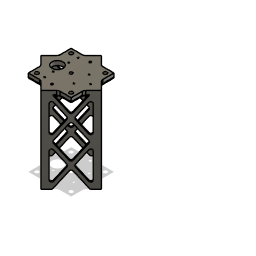
sensors-plate_lidar3d_generic-support (Autodesk Fusion 360 design; units mm, degrees)
Autodesk Fusion 360 part; units mm, degrees
note: some values were not read from the file. Set by a fixed rule: which sketch regions a step uses.
ref_plane "WorkPlane1" through (176, 592, -131) normal (0, 1, 0) x (-1, 0, 0)
sketch "Sketch4" plane through (0, 592, 0) normal (0, 1, 0) x (1, 0, 0)
  line L0 (178, -131) -> (180, -131)
  line L1 (176, 131) -> (178, 131)
  line L2 (176, -131) -> (178, -131)
  line L3 (178, 131) -> (180, 131)
  line L4 (180, -131) -> (180, 131)
  line L5 (176, 133) -> (176, 135)
  line L6 (-176, 131) -> (-176, 133)
  line L7 (176, 131) -> (176, 133)
  line L8 (-176, 133) -> (-176, 135)
  line L9 (176, 135) -> (-176, 135)
  line L10 (-176, -133) -> (-176, -135)
  line L11 (176, -131) -> (176, -133)
  line L12 (-176, -131) -> (-176, -133)
  line L13 (176, -133) -> (176, -135)
  line L14 (-176, -135) -> (176, -135)
  line L15 (-178, 131) -> (-180, 131)
  line L16 (-176, -131) -> (-178, -131)
  line L17 (-176, 131) -> (-178, 131)
  line L18 (-178, -131) -> (-180, -131)
  line L19 (-180, 131) -> (-180, -131)
  circle A0 centre (-120, 60) radius 2 construction
  circle A1 centre (0, -120) radius 2 construction
  circle A2 centre (-120, -120) radius 2 construction
  circle A3 centre (120, 0) radius 2 construction
  circle A4 centre (0, 120) radius 2 construction
  circle A5 centre (0, 60) radius 2 construction
  circle A6 centre (-165.5, -26.5835) radius 2.5
  circle A7 centre (0, 0) radius 2 construction
  circle A8 centre (-60, -120) radius 2 construction
  circle A9 centre (165.5, 26.5835) radius 2.5
  circle A10 centre (-165.5, -78.1855) radius 2.5
  circle A11 centre (-120, 0) radius 2 construction
  circle A12 centre (-120, 120) radius 2 construction
  circle A13 centre (60, -60) radius 2 construction
  circle A14 centre (60, -120) radius 2 construction
  circle A15 centre (120, 60) radius 2 construction
  circle A16 centre (-60, -60) radius 2 construction
  circle A17 centre (0, -60) radius 2 construction
  circle A18 centre (-165.5, 26.5835) radius 2.5
  circle A19 centre (-60, 60) radius 2 construction
  circle A20 centre (165.5, -26.5835) radius 2.5
  circle A21 centre (-60, 0) radius 2 construction
  circle A22 centre (-120, -60) radius 2 construction
  circle A23 centre (-165.5, 78.1855) radius 2.5
  circle A24 centre (120, -60) radius 2 construction
  circle A25 centre (120, -120) radius 2 construction
  circle A26 centre (60, 120) radius 2 construction
  circle A27 centre (165.5, -78.1855) radius 2.5
  circle A28 centre (120, 120) radius 2 construction
  circle A29 centre (60, 0) radius 2 construction
  circle A30 centre (-60, 120) radius 2 construction
  circle A31 centre (165.5, 78.1855) radius 2.5
  circle A32 centre (60, 60) radius 2 construction
  line L20 (0, 70.7107) -> (-70.7107, 0)
  line L21 (-70.7107, 0) -> (0, -70.7107)
  line L22 (0, -70.7107) -> (70.7107, 0)
  line L23 (70.7107, 0) -> (0, 70.7107)
  line L24 (-180, 0) -> (180, 0) construction
  dimension "d323" = 50
  dimension "d324" = 135
  constraint coincident A7.centre origin
  constraint midpoint L19 L24.start
  constraint midpoint L4 L24.end
  measures "d323" distance of A7.centre L23
  measures "d324" angle of L23 L24
extrude "Extrude2" add sketch "Sketch4" against normal blind 8 contours L20 L21 L22 L23
sketch "Sketch6" plane through (0, 584, 0) normal (0, -1, 0) x (1, 0, 0)
  line L0 (0, -70.7107) -> (70.7107, 0)
  line L1 (70.7107, 0) -> (0, 70.7107)
  line L2 (0, 70.7107) -> (-70.7107, 0)
  line L3 (-70.7107, 0) -> (0, -70.7107)
  line L4 (180, -131) -> (180, 131)
  line L5 (180, -131) -> (176, -131)
  line L6 (176, 131) -> (180, 131)
  line L7 (-176, -135) -> (176, -135)
  line L8 (-176, -135) -> (-176, -131)
  line L9 (176, -131) -> (176, -135)
  line L10 (176, 135) -> (-176, 135)
  line L11 (176, 135) -> (176, 131)
  line L12 (-176, 131) -> (-176, 135)
  line L13 (-180, 131) -> (-180, -131)
  line L14 (-180, 131) -> (-176, 131)
  line L15 (-176, -131) -> (-180, -131)
  circle A0 centre (-120, -60) radius 2
  circle A1 centre (0, 120) radius 2
  circle A2 centre (-120, 120) radius 2
  circle A3 centre (120, 0) radius 2
  circle A4 centre (0, -120) radius 2
  circle A5 centre (0, -60) radius 2 construction
  circle A6 centre (-165.5, 26.5835) radius 2.5
  circle A7 centre (0, 0) radius 2 construction
  circle A8 centre (-60, 120) radius 2
  circle A9 centre (165.5, -26.5835) radius 2.5
  circle A10 centre (-165.5, 78.1855) radius 2.5
  circle A11 centre (-120, 0) radius 2
  circle A12 centre (-120, -120) radius 2
  circle A13 centre (60, 60) radius 2
  circle A14 centre (60, 120) radius 2
  circle A15 centre (120, -60) radius 2
  circle A16 centre (-60, 60) radius 2
  circle A17 centre (0, 60) radius 2 construction
  circle A18 centre (-165.5, -26.5835) radius 2.5
  circle A19 centre (-60, -60) radius 2
  circle A20 centre (165.5, 26.5835) radius 2.5
  circle A21 centre (-60, 0) radius 2 construction
  circle A22 centre (-120, 60) radius 2
  circle A23 centre (-165.5, -78.1855) radius 2.5
  circle A24 centre (120, 60) radius 2
  circle A25 centre (120, 120) radius 2
  circle A26 centre (60, -120) radius 2
  circle A27 centre (165.5, 78.1855) radius 2.5
  circle A28 centre (120, -120) radius 2
  circle A29 centre (60, 0) radius 2 construction
  circle A30 centre (-60, -120) radius 2
  circle A31 centre (165.5, -78.1855) radius 2.5
  circle A32 centre (60, -60) radius 2
  line L16 (45, 0) -> (-22.5, 38.9711) construction
  line L17 (-22.5, 38.9711) -> (-22.5, -38.9711) construction
  line L18 (-22.5, -38.9711) -> (45, 0) construction
  line L19 (45, 0) -> (-22.5, 0) construction
  line L20 (-70.7107, 0) -> (70.7107, 0) construction
  line L21 (0, 70.7107) -> (0, -70.7107) construction
  circle A33 centre (-22.5, 38.9711) radius 1.65
  circle A34 centre (45, 0) radius 1.65
  circle A35 centre (-22.5, -38.9711) radius 1.65
  line L22 (40, 40) -> (-40, 40) construction
  line L23 (-40, 40) -> (-40, -40) construction
  line L24 (-40, -40) -> (40, -40) construction
  line L25 (40, -40) -> (40, 40) construction
  circle A36 centre (-40, 40) radius 4.15
  circle A37 centre (40, 40) radius 4.15
  circle A38 centre (40, -40) radius 4.15
  circle A39 centre (-40, -40) radius 4.15
  line L26 (50, 50) -> (-50, 50)
  line L27 (-50, 50) -> (-50, -50)
  line L28 (-50, -50) -> (50, -50)
  line L29 (50, -50) -> (50, 50)
  circle A40 centre (-24, 18) radius 1.65
  circle A41 centre (24, 18) radius 1.65
  circle A42 centre (24, -18) radius 1.65
  circle A43 centre (-24, -18) radius 1.65
  circle A44 centre (0, 0) radius 3.325
  circle A45 centre (0, 44.45) radius 2.15
  circle A46 centre (0, -44.45) radius 2.15
  circle A47 centre (0, 0) radius 45 construction
  circle A48 centre (0, -45) radius 2.15
  circle A49 centre (0, 45) radius 2.15
  line L30 (-2.15, -44.45) -> (-2.15, -45)
  line L31 (2.15, -44.45) -> (2.15, -45)
  line L32 (-2.15, 44.45) -> (-2.15, 45)
  line L33 (2.15, 45) -> (2.15, 44.45)
  circle A50 centre (0, 0) radius 24 construction
  circle A51 centre (0, 0) radius 40 construction
  circle A52 centre (-32, 0) radius 8 construction
  circle A53 centre (-32, 0) radius 13
  line L34 (-60, 0) -> (0, 60) construction
  line L35 (0, 60) -> (60, 0) construction
  line L36 (60, 0) -> (0, -60) construction
  line L37 (0, -60) -> (-60, 0) construction
  line L38 (-51.5147, 0) -> (0, 51.5147) construction
  line L39 (0, 51.5147) -> (51.5147, 0) construction
  line L40 (51.5147, 0) -> (0, -51.5147) construction
  line L41 (0, -51.5147) -> (-51.5147, 0) construction
  line L42 (-51.5147, 0) -> (-61.1127, 9.598)
  line L43 (-51.5147, 0) -> (-61.1127, -9.598)
  line L44 (0, 51.5147) -> (9.598, 61.1127)
  line L45 (0, 51.5147) -> (-9.598, 61.1127)
  line L46 (0, -51.5147) -> (-9.598, -61.1127)
  line L47 (0, -51.5147) -> (9.598, -61.1127)
  line L48 (51.5147, 0) -> (61.1127, -9.598)
  line L49 (51.5147, 0) -> (61.1127, 9.598)
  dimension "d331" = 45
  dimension "d332" = 3.3
  dimension "d333" = 40
  dimension "d334" = 135
  dimension "d335" = 8.3
  dimension "d336" = 50
  dimension "d338" = 3.3
  dimension "d339" = 6.65
  dimension "d340" = 4.3
  dimension "d341" = 88.9
  dimension "d536" = 48
  dimension "d537" = 80
  dimension "d538" = 5
  dimension "d539" = 24
  dimension "d540" = 18
  dimension "d545" = 6
  constraint coincident A7.centre A44.centre
  constraint midpoint L17 L19.end
  constraint coincident L2.end L3.start
  constraint coincident L0.end L1.start
  constraint coincident L1.end L2.start
  constraint coincident L0.start L3.end
  constraint collinear L19 L20
  constraint coincident L16.end L17.start
  constraint coincident L16.start L18.end
  constraint coincident L17.end L18.start
  constraint equal A33 A35
  constraint equal A33 A34
  constraint coincident L22.end L23.start
  constraint coincident L22.start L25.end
  constraint coincident L24.end L25.start
  constraint coincident L23.end L24.start
  constraint equal A36 A39
  constraint equal A36 A38
  constraint equal A36 A37
  constraint parallel L25 L29
  constraint equal A40 A43
  constraint equal A40 A41
  constraint equal A40 A42
  constraint coincident L21 A45.centre
  constraint coincident L21 A46.centre
  constraint symmetric L20 A45 A46
  constraint coincident L16.start A47
  constraint coincident L21 A48.centre
  constraint coincident A47 A48.centre
  constraint coincident A47 A49.centre
  constraint coincident L21 A49.centre
  constraint equal A45 A49
  constraint equal A45 A48
  constraint coincident A46 L30.start
  constraint coincident A48 L30.end
  constraint coincident A46 L31.start
  constraint coincident A48 L31.end
  constraint tangent A46 L30
  constraint tangent A48 L30
  constraint tangent A46 L31
  constraint tangent A48 L31
  constraint coincident A45 L32.start
  constraint coincident A49 L32.end
  constraint coincident A49 L33.start
  constraint coincident A45 L33.end
  constraint tangent A49 L33
  constraint tangent A45 L33
  constraint tangent A49 L32
  constraint tangent A45 L32
  constraint concentric A44 A50
  constraint tangent A50 A52
  constraint tangent A51 A52
  constraint coincident L20 A52.centre
  constraint symmetric L21 A40 A41
  constraint symmetric L20 A40 A43
  constraint symmetric L20 A41 A42
  constraint coincident A21.centre L34.start
  constraint coincident A17.centre L34.end
  constraint coincident A29.centre L35.end
  constraint coincident A5.centre L36.end
  constraint coincident L2 L42.end
  constraint perpendicular L2 L42
  constraint coincident L3 L43.end
  constraint perpendicular L3 L43
  constraint coincident L1 L44.end
  constraint perpendicular L1 L44
  constraint coincident L2 L45.end
  constraint perpendicular L2 L45
  constraint coincident L3 L46.end
  constraint perpendicular L3 L46
  constraint coincident L0 L47.end
  constraint perpendicular L0 L47
  constraint coincident L0 L48.end
  constraint perpendicular L0 L48
  constraint coincident L1 L49.end
  constraint perpendicular L1 L49
  measures "d331" distance of L16.start A7.centre
  measures "d332" diameter of A33
  measures "d333" distance of A7.centre L25
  measures "d334" angle of L1 L25
  measures "d335" diameter of A36
  measures "d336" distance of A7.centre L29
  measures "d338" diameter of A40
  measures "d339" diameter of A44
  measures "d340" diameter of A45
  measures "d341" distance of A45.centre A46.centre
  measures "d536" diameter of A50
  measures "d537" diameter of A51
  measures "d539" distance of L21 A41.centre
  measures "d540" distance of L20 A41.centre
extrude "Extrude3" cut sketch "Sketch6" against normal up to surface (8 mm away) contours A33 | A34 | A35 | A40 | A41 | A42 | A43 | A44 | A45 A49 | A45 A49 L32 | A45 A49 L33 | A45 A49 | A45 A49 | A46 A48 | A46 A48 L31 | A46 A48 L30 | A46 A48 | A46 A48 | A53
extrude "Extrude4" add sketch "Sketch6" against normal up to surface (8 mm away) contours L0 L28 L29 | L3 L27 L28 | L1 L26 L29 | L2 L26 L27
extrude "Extrude5" add sketch "Sketch6" along normal up to surface (192 mm away) contours L0 L3 L46 L47 | L0 L1 L48 L49 | L2 L3 L42 L43 | L1 L2 L44 L45
sketch "Sketch7" plane through (-35.3553, 0, -35.3553) normal (-0.707107, 0, -0.707107) x (-0.707107, 0, 0.707107)
  line L0 (20.7107, 592) -> (20.7107, 584)
  line L1 (20.7107, 584) -> (36.4264, 584)
  line L2 (36.4264, 584) -> (36.4264, 392)
  line L3 (36.4264, 392) -> (50, 392)
  line L4 (50, 392) -> (50, 592)
  line L5 (50, 592) -> (20.7107, 592)
  line L6 (-20.7107, 584) -> (-20.7107, 592)
  line L7 (-20.7107, 592) -> (-50, 592)
  line L8 (-50, 592) -> (-50, 392)
  line L9 (-50, 392) -> (-36.4264, 392)
  line L10 (-36.4264, 392) -> (-36.4264, 584)
  line L11 (-36.4264, 584) -> (-20.7107, 584)
  line L12 (36.4264, 584) -> (-36.4264, 488) construction
  line L13 (-36.4264, 488) -> (36.4264, 392) construction
  line L14 (-36.4264, 392) -> (36.4264, 488) construction
  line L15 (36.4264, 488) -> (-36.4264, 584) construction
  line L16 (-33.24, 389.5819) -> (41.4478, 488)
  line L17 (41.4478, 488) -> (-33.24, 586.4181)
  line L18 (-39.6128, 394.4181) -> (31.405, 488)
  line L19 (31.405, 488) -> (-39.6128, 581.5819)
  line L20 (33.24, 586.4181) -> (-41.4478, 488)
  line L21 (-41.4478, 488) -> (33.24, 389.5819)
  line L22 (39.6128, 581.5819) -> (-31.405, 488)
  line L23 (-31.405, 488) -> (39.6128, 394.4181)
  line L24 (36.4264, 392) -> (-36.4264, 392)
  dimension "d549" = 4
  dimension "d550" = -4
  dimension "d551" = 4
  dimension "d552" = -4
  constraint coincident L1.end L2.start
  constraint midpoint L10 L12.end
  constraint coincident L2.end L3.start
  constraint coincident L9.end L10.start
  constraint midpoint L2 L14.end
  constraint coincident L10.end L11.start
extrude "Extrude6" add sketch "Sketch7" against normal blind 4 contours L1 L2 L17 L20 L22 | L10 L11 L17 L19 L20 | L17 L19 L20 L22 | L2 L16 L21 L23 L24 | L2 L16 L17 L18 L19 L22 L23 | L10 L18 L19 L20 L21 L22 L23 | L16 L18 L21 L23 | L10 L16 L18 L21 L24
sketch "Sketch8" plane through (35.3553, 0, 35.3553) normal (0.707107, 0, 0.707107) x (0.707107, 0, -0.707107)
  line L0 (-20.7107, 584) -> (-20.7107, 592)
  line L1 (-20.7107, 592) -> (-50, 592)
  line L2 (-50, 592) -> (-50, 392)
  line L3 (-50, 392) -> (-36.4264, 392)
  line L4 (-36.4264, 392) -> (-36.4264, 584)
  line L5 (-36.4264, 584) -> (-20.7107, 584)
  line L6 (31.405, 488) -> (0, 446.6168)
  line L7 (0, 446.6168) -> (-31.405, 488)
  line L8 (-31.405, 488) -> (0, 529.3832)
  line L9 (0, 529.3832) -> (31.405, 488)
  line L10 (-36.4264, 481.3832) -> (-5.0214, 440)
  line L11 (-5.0214, 440) -> (-36.4264, 398.6168)
  line L12 (-36.4264, 398.6168) -> (-36.4264, 392)
  line L13 (-36.4264, 392) -> (-31.405, 392)
  line L14 (-31.405, 392) -> (0, 433.3832)
  line L15 (0, 433.3832) -> (31.405, 392)
  line L16 (31.405, 392) -> (36.4264, 392)
  line L17 (36.4264, 392) -> (36.4264, 398.6168)
  line L18 (36.4264, 398.6168) -> (5.0214, 440)
  line L19 (5.0214, 440) -> (36.4264, 481.3832)
  line L20 (36.4264, 481.3832) -> (36.4264, 494.6168)
  line L21 (36.4264, 494.6168) -> (5.0214, 536)
  line L22 (5.0214, 536) -> (36.4264, 577.3832)
  line L23 (36.4264, 577.3832) -> (36.4264, 584)
  line L24 (36.4264, 584) -> (31.405, 584)
  line L25 (31.405, 584) -> (0, 542.6168)
  line L26 (0, 542.6168) -> (-31.405, 584)
  line L27 (-31.405, 584) -> (-36.4264, 584)
  line L28 (-36.4264, 584) -> (-36.4264, 577.3832)
  line L29 (-36.4264, 577.3832) -> (-5.0214, 536)
  line L30 (-5.0214, 536) -> (-36.4264, 494.6168)
  line L31 (-36.4264, 494.6168) -> (-36.4264, 481.3832)
extrude "Extrude7" add sketch "Sketch8" against normal blind 4 contours L4 L5 L10 L11 L12 L13 L14 L15 L16 L17 L18 L19 L20 L21 L22 L23 L24 L25 L26 L27 L28 L29 L30 L31
sketch "Sketch9" plane through (-35.3553, 0, 35.3553) normal (-0.707107, 0, 0.707107) x (0.707107, 0, 0.707107)
  line L0 (-20.7107, 584) -> (-20.7107, 592)
  line L1 (-20.7107, 592) -> (-50, 592)
  line L2 (-50, 592) -> (-50, 392)
  line L3 (-50, 392) -> (-36.4264, 392)
  line L4 (-36.4264, 392) -> (-36.4264, 584)
  line L5 (-36.4264, 584) -> (-20.7107, 584)
  line L6 (20.7107, 592) -> (20.7107, 584)
  line L7 (20.7107, 584) -> (36.4264, 584)
  line L8 (36.4264, 584) -> (36.4264, 392)
  line L9 (36.4264, 392) -> (50, 392)
  line L10 (50, 392) -> (50, 592)
  line L11 (50, 592) -> (20.7107, 592)
  line L12 (-36.4264, 584) -> (36.4264, 488) construction
  line L13 (36.4264, 488) -> (-36.4264, 392) construction
  line L14 (36.4264, 392) -> (-36.4264, 488) construction
  line L15 (-36.4264, 488) -> (36.4264, 584) construction
  line L16 (39.6128, 394.4181) -> (-31.405, 488)
  line L17 (-31.405, 488) -> (39.6128, 581.5819)
  line L18 (33.24, 389.5819) -> (-41.4478, 488)
  line L19 (-41.4478, 488) -> (33.24, 586.4181)
  line L20 (-39.6128, 581.5819) -> (31.405, 488)
  line L21 (31.405, 488) -> (-39.6128, 394.4181)
  line L22 (-33.24, 586.4181) -> (41.4478, 488)
  line L23 (41.4478, 488) -> (-33.24, 389.5819)
  line L24 (36.4264, 392) -> (-36.4264, 392)
  dimension "d557" = 4
  dimension "d558" = -4
  dimension "d559" = 4
  dimension "d560" = -4
  constraint coincident L4.end L5.start
  constraint midpoint L8 L12.end
  constraint coincident L3.end L4.start
  constraint coincident L8.end L9.start
  constraint midpoint L4 L14.end
  constraint coincident L7.end L8.start
extrude "Extrude8" add sketch "Sketch9" against normal blind 4 contours L4 L5 L19 L20 L22 | L17 L19 L20 L22 | L7 L8 L17 L19 L22 | L4 L16 L17 L18 L19 L20 L21 | L8 L16 L17 L20 L21 L22 L23 | L4 L18 L21 L23 L24 | L16 L18 L21 L23 | L8 L16 L18 L23 L24
sketch "Sketch10" plane through (35.3553, 0, -35.3553) normal (0.707107, 0, -0.707107) x (-0.707107, 0, -0.707107)
  line L0 (-20.7107, 584) -> (-20.7107, 592)
  line L1 (-20.7107, 592) -> (-50, 592)
  line L2 (-50, 592) -> (-50, 392)
  line L3 (-50, 392) -> (-36.4264, 392)
  line L4 (-36.4264, 392) -> (-36.4264, 584)
  line L5 (-36.4264, 584) -> (-20.7107, 584)
  line L6 (-31.405, 488) -> (0, 529.3832)
  line L7 (0, 529.3832) -> (31.405, 488)
  line L8 (31.405, 488) -> (0, 446.6168)
  line L9 (0, 446.6168) -> (-31.405, 488)
  line L10 (-5.0214, 440) -> (-36.4264, 398.6168)
  line L11 (-36.4264, 398.6168) -> (-36.4264, 392)
  line L12 (-36.4264, 392) -> (-31.405, 392)
  line L13 (-31.405, 392) -> (0, 433.3832)
  line L14 (0, 433.3832) -> (31.405, 392)
  line L15 (31.405, 392) -> (36.4264, 392)
  line L16 (36.4264, 392) -> (36.4264, 398.6168)
  line L17 (36.4264, 398.6168) -> (5.0214, 440)
  line L18 (5.0214, 440) -> (36.4264, 481.3832)
  line L19 (36.4264, 481.3832) -> (36.4264, 494.6168)
  line L20 (36.4264, 494.6168) -> (5.0214, 536)
  line L21 (5.0214, 536) -> (36.4264, 577.3832)
  line L22 (36.4264, 577.3832) -> (36.4264, 584)
  line L23 (36.4264, 584) -> (31.405, 584)
  line L24 (31.405, 584) -> (0, 542.6168)
  line L25 (0, 542.6168) -> (-31.405, 584)
  line L26 (-31.405, 584) -> (-36.4264, 584)
  line L27 (-36.4264, 584) -> (-36.4264, 577.3832)
  line L28 (-36.4264, 577.3832) -> (-5.0214, 536)
  line L29 (-5.0214, 536) -> (-36.4264, 494.6168)
  line L30 (-36.4264, 494.6168) -> (-36.4264, 481.3832)
  line L31 (-36.4264, 481.3832) -> (-5.0214, 440)
extrude "Extrude9" add sketch "Sketch10" against normal blind 4 contours L4 L5 L10 L11 L12 L13 L14 L15 L16 L17 L18 L19 L20 L21 L22 L23 L24 L25 L26 L27 L28 L29 L30 L31
sketch "Sketch11" plane through (0, 392, 0) normal (0, -1, 0) x (1, 0, 0)
  line L0 (0, -51.5147) -> (-6.7696, -58.2843)
  line L1 (-6.7696, -58.2843) -> (-10.3202, -54.7336)
  line L2 (-10.3202, -54.7336) -> (-13.1486, -57.562)
  line L3 (-13.1486, -57.562) -> (0, -70.7107)
  line L4 (0, -70.7107) -> (13.1486, -57.562)
  line L5 (13.1486, -57.562) -> (10.3202, -54.7336)
  line L6 (10.3202, -54.7336) -> (6.7696, -58.2843)
  line L7 (6.7696, -58.2843) -> (0, -51.5147)
  circle A0 centre (-120, -60) radius 2
  circle A1 centre (0, 120) radius 2
  circle A2 centre (-120, 120) radius 2
  circle A3 centre (120, 0) radius 2
  circle A4 centre (0, -120) radius 2
  circle A5 centre (0, -60) radius 2 construction
  circle A6 centre (-165.5, 26.5835) radius 2.5
  circle A7 centre (0, 0) radius 2
  circle A8 centre (-60, 120) radius 2
  circle A9 centre (165.5, -26.5835) radius 2.5
  circle A10 centre (-165.5, 78.1855) radius 2.5
  circle A11 centre (-120, 0) radius 2
  circle A12 centre (-120, -120) radius 2
  circle A13 centre (60, 60) radius 2
  circle A14 centre (60, 120) radius 2
  circle A15 centre (120, -60) radius 2
  circle A16 centre (-60, 60) radius 2
  circle A17 centre (0, 60) radius 2 construction
  circle A18 centre (-165.5, -26.5835) radius 2.5
  circle A19 centre (-60, -60) radius 2
  circle A20 centre (165.5, 26.5835) radius 2.5
  circle A21 centre (-60, 0) radius 2 construction
  circle A22 centre (-120, 60) radius 2
  circle A23 centre (-165.5, -78.1855) radius 2.5
  circle A24 centre (120, 60) radius 2
  circle A25 centre (120, 120) radius 2
  circle A26 centre (60, -120) radius 2
  circle A27 centre (165.5, 78.1855) radius 2.5
  circle A28 centre (120, -120) radius 2
  circle A29 centre (60, 0) radius 2 construction
  circle A30 centre (-60, -120) radius 2
  circle A31 centre (165.5, -78.1855) radius 2.5
  circle A32 centre (60, -60) radius 2
  line L8 (176, 131) -> (176, -131)
  line L9 (176, -131) -> (-176, -131)
  line L10 (-176, -131) -> (-176, 131)
  line L11 (-176, 131) -> (176, 131)
  circle A33 centre (0, -60) radius 1.4
  circle A34 centre (-60, 0) radius 1.4
  circle A35 centre (0, 60) radius 1.4
  circle A36 centre (60, 0) radius 1.4
  dimension "d565" = 2.8
  constraint concentric A5 A33
  constraint concentric A21 A34
  constraint concentric A17 A35
  constraint concentric A29 A36
  constraint equal A34 A36
  constraint equal A33 A36
  constraint equal A35 A36
  measures "d565" diameter of A36
extrude "Extrude10" cut sketch "Sketch11" against normal blind 50 contours A33 | A34 | A35 | A36
hole "Hole1" at (-24, 584, -18) direction (0, 1, 0) diameter 3 depth 8 tip angle 180 countersink diameter 6 countersink angle 90
hole "Hole2" at (24, 584, -18) direction (0, 1, 0) diameter 3 depth 8 tip angle 180 countersink diameter 6 countersink angle 90
hole "Hole3" at (24, 584, 18) direction (0, 1, 0) diameter 3 depth 8 tip angle 180 countersink diameter 6 countersink angle 90
hole "Hole4" at (-24, 584, 18) direction (0, 1, 0) diameter 3 depth 8 tip angle 180 countersink diameter 6 countersink angle 90
hole "Hole5" at (-22.5, 584, -38.9711) direction (0, 1, 0) diameter 3 depth 8 tip angle 180 countersink diameter 6 countersink angle 90
hole "Hole6" at (45, 584, 0) direction (0, 1, 0) diameter 3 depth 8 tip angle 180 countersink diameter 6 countersink angle 90
hole "Hole7" at (-22.5, 584, 38.9711) direction (0, 1, 0) diameter 3 depth 8 tip angle 180 countersink diameter 6 countersink angle 90
sketch "Sketch13" plane through (0, 584, 0) normal (0, -1, 0) x (1, 0, 0)
  circle A0 centre (-22.5, 38.9711) radius 3
  circle A1 centre (45, 0) radius 3
  circle A2 centre (-22.5, -38.9711) radius 3
  circle A3 centre (-24, 18) radius 3
  circle A4 centre (24, 18) radius 3
  circle A5 centre (24, -18) radius 3
  circle A6 centre (-24, -18) radius 3
  line L0 (10.3202, -54.7336) -> (13.1486, -57.562)
  line L1 (13.1486, -57.562) -> (20.7107, -50)
  line L2 (20.7107, -50) -> (50, -50)
  line L3 (50, -50) -> (50, -20.7107)
  line L4 (50, -20.7107) -> (57.562, -13.1486)
  line L5 (57.562, -13.1486) -> (54.7336, -10.3202)
  line L6 (54.7336, -10.3202) -> (58.2843, -6.7696)
  line L7 (58.2843, -6.7696) -> (51.5147, 0)
  line L8 (51.5147, 0) -> (58.2843, 6.7696)
  line L9 (58.2843, 6.7696) -> (54.7336, 10.3202)
  line L10 (54.7336, 10.3202) -> (57.562, 13.1486)
  line L11 (57.562, 13.1486) -> (50, 20.7107)
  line L12 (50, 20.7107) -> (50, 50)
  line L13 (50, 50) -> (20.7107, 50)
  line L14 (20.7107, 50) -> (13.1486, 57.562)
  line L15 (13.1486, 57.562) -> (10.3202, 54.7336)
  line L16 (10.3202, 54.7336) -> (6.7696, 58.2843)
  line L17 (6.7696, 58.2843) -> (0, 51.5147)
  line L18 (0, 51.5147) -> (-6.7696, 58.2843)
  line L19 (-6.7696, 58.2843) -> (-10.3202, 54.7336)
  line L20 (-10.3202, 54.7336) -> (-13.1486, 57.562)
  line L21 (-13.1486, 57.562) -> (-20.7107, 50)
  line L22 (-20.7107, 50) -> (-50, 50)
  line L23 (-50, 50) -> (-50, 20.7107)
  line L24 (-50, 20.7107) -> (-57.562, 13.1486)
  line L25 (-57.562, 13.1486) -> (-54.7336, 10.3202)
  line L26 (-54.7336, 10.3202) -> (-58.2843, 6.7696)
  line L27 (-58.2843, 6.7696) -> (-51.5147, 0)
  line L28 (-51.5147, 0) -> (-58.2843, -6.7696)
  line L29 (-58.2843, -6.7696) -> (-54.7336, -10.3202)
  line L30 (-54.7336, -10.3202) -> (-57.562, -13.1486)
  line L31 (-57.562, -13.1486) -> (-50, -20.7107)
  line L32 (-50, -20.7107) -> (-50, -50)
  line L33 (-50, -50) -> (-20.7107, -50)
  line L34 (-20.7107, -50) -> (-13.1486, -57.562)
  line L35 (-13.1486, -57.562) -> (-10.3202, -54.7336)
  line L36 (-10.3202, -54.7336) -> (-6.7696, -58.2843)
  line L37 (-6.7696, -58.2843) -> (0, -51.5147)
  line L38 (0, -51.5147) -> (6.7696, -58.2843)
  line L39 (6.7696, -58.2843) -> (10.3202, -54.7336)
  circle A7 centre (40, 40) radius 4.15
  circle A8 centre (-40, 40) radius 4.15
  circle A9 centre (40, -40) radius 4.15
  circle A10 centre (-40, -40) radius 4.15
  circle A11 centre (0, 0) radius 3.325
  circle A12 centre (-32, 0) radius 13
  arc A13 (2.15, -44.45) -> (-2.15, -44.45) centre (0, -44.45) ccw
  line L40 (2.15, -44.45) -> (2.15, -45)
  arc A14 (-2.15, -45) -> (2.15, -45) centre (0, -45) ccw
  line L41 (-2.15, -45) -> (-2.15, -44.45)
  line L42 (-2.15, 44.45) -> (-2.15, 45)
  arc A15 (2.15, 45) -> (-2.15, 45) centre (0, 45) ccw
  line L43 (2.15, 45) -> (2.15, 44.45)
  arc A16 (-2.15, 44.45) -> (2.15, 44.45) centre (0, 44.45) ccw
  line L44 (-20.7107, -50) -> (50, 20.7107) construction
  line L45 (20.7107, 50) -> (-50, -20.7107) construction
  line L46 (50, -20.7107) -> (-20.7107, 50) construction
  line L47 (20.7107, -50) -> (-50, 20.7107) construction
  circle A17 centre (-32, 0) radius 15
  line L48 (-51.5147, 0) -> (51.5147, 0) construction
  line L49 (0, -51.5147) -> (0, 51.5147) construction
  line L50 (22.1249, -50) -> (-50, 22.1249)
  line L51 (-50.7071, 20.0036) -> (20.0036, -50.7071)
  line L52 (50, -50) -> (-50, 50) construction
  line L53 (-50, -50) -> (50, 50) construction
  line L54 (-20.0036, 50.7071) -> (50.7071, -20.0036)
  line L55 (50, -22.1249) -> (-22.1249, 50)
  line L56 (-20.0036, -50.7071) -> (50.7071, 20.0036)
  line L57 (-22.1249, -50) -> (50, 22.1249)
  line L58 (-50.7071, -20.0036) -> (20.0036, 50.7071)
  line L59 (-50, -22.1249) -> (22.1249, 50)
  line L60 (20.2965, 49) -> (13.1486, 56.1478)
  line L61 (13.1486, 56.1478) -> (10.3202, 53.3194)
  line L62 (10.3202, 53.3194) -> (6.7696, 56.8701)
  line L63 (6.7696, 56.8701) -> (0, 50.1005)
  line L64 (0, 50.1005) -> (-6.7696, 56.8701)
  line L65 (-6.7696, 56.8701) -> (-10.3202, 53.3194)
  line L66 (-10.3202, 53.3194) -> (-13.1486, 56.1478)
  line L67 (-13.1486, 56.1478) -> (-20.2965, 49)
  line L68 (-20.2965, 49) -> (-49, 49)
  line L69 (-49, 49) -> (-49, 20.2965)
  line L70 (-49, 20.2965) -> (-56.1478, 13.1486)
  line L71 (-56.1478, 13.1486) -> (-53.3194, 10.3202)
  line L72 (-53.3194, 10.3202) -> (-56.8701, 6.7696)
  line L73 (-56.8701, 6.7696) -> (-50.1005, 0)
  line L74 (-50.1005, 0) -> (-56.8701, -6.7696)
  line L75 (-56.8701, -6.7696) -> (-53.3194, -10.3202)
  line L76 (-53.3194, -10.3202) -> (-56.1478, -13.1486)
  line L77 (-56.1478, -13.1486) -> (-49, -20.2965)
  line L78 (-49, -20.2965) -> (-49, -49)
  line L79 (-49, -49) -> (-20.2965, -49)
  line L80 (-20.2965, -49) -> (-13.1486, -56.1478)
  line L81 (-13.1486, -56.1478) -> (-10.3202, -53.3194)
  line L82 (-10.3202, -53.3194) -> (-6.7696, -56.8701)
  line L83 (-6.7696, -56.8701) -> (0, -50.1005)
  line L84 (0, -50.1005) -> (6.7696, -56.8701)
  line L85 (6.7696, -56.8701) -> (10.3202, -53.3194)
  line L86 (10.3202, -53.3194) -> (13.1486, -56.1478)
  line L87 (13.1486, -56.1478) -> (20.2965, -49)
  line L88 (20.2965, -49) -> (49, -49)
  line L89 (49, -49) -> (49, -20.2965)
  line L90 (49, -20.2965) -> (56.1478, -13.1486)
  line L91 (56.1478, -13.1486) -> (53.3194, -10.3202)
  line L92 (53.3194, -10.3202) -> (56.8701, -6.7696)
  line L93 (56.8701, -6.7696) -> (50.1005, 0)
  line L94 (50.1005, 0) -> (56.8701, 6.7696)
  line L95 (56.8701, 6.7696) -> (53.3194, 10.3202)
  line L96 (53.3194, 10.3202) -> (56.1478, 13.1486)
  line L97 (56.1478, 13.1486) -> (49, 20.2965)
  line L98 (49, 20.2965) -> (49, 49)
  line L99 (49, 49) -> (20.2965, 49)
  dimension "d604" = 2
  dimension "d605" = 1
  dimension "d606" = 1
  dimension "d607" = 1
  dimension "d608" = 1
  dimension "d609" = -1
  constraint coincident L33.end L34.start
  constraint coincident L11.end L12.start
  constraint coincident L13.end L14.start
  constraint coincident L31.end L32.start
  constraint coincident L3.end L4.start
  constraint coincident L21.end L22.start
  constraint coincident L1.end L2.start
  constraint coincident L23.end L24.start
  constraint coincident L27.end L28.start
  constraint coincident L7.end L8.start
  constraint coincident L37.end L38.start
  constraint coincident L17.end L18.start
  constraint coincident L2 L50.start
  constraint coincident L23 L50.end
  constraint parallel L47 L50
  constraint coincident L24 L51.start
  constraint coincident L1 L51.end
  constraint parallel L47 L51
  constraint coincident L2.end L3.start
  constraint coincident L22.end L23.start
  constraint coincident L32.end L33.start
  constraint coincident L12.end L13.start
  constraint symmetric L50.start L52 L55.start
  constraint symmetric L50.end L52 L55.end
  constraint symmetric L51.start L52 L54.start
  constraint symmetric L51.end L52 L54.end
  constraint coincident L34 L56.start
  constraint coincident L11 L56.end
  constraint coincident L33 L57.start
  constraint coincident L12 L57.end
  constraint parallel L44 L57
  constraint parallel L44 L56
  constraint symmetric L53 L56.start L58.start
  constraint symmetric L53 L56.end L58.end
  constraint symmetric L53 L57.start L59.start
  constraint symmetric L53 L57.end L59.end
  measures "d605" distance of L47 L50
  measures "d606" distance of L47 L51
  measures "d607" distance of L44 L56
  measures "d608" distance of L44 L57
extrude "Extrude11" add sketch "Sketch13" along normal blind 2 contours L0 L1 L34 L35 L36 L37 L38 L39 L51 L56 L80 L81 L82 L83 L84 L85 L86 L87 | L1 L2 L50 L51 L87 L88 | L50 L51 L56 L87 L88 | L2 L3 L50 L55 L88 L89 | L51 L56 L57 L79 L80 | L50 L51 L56 L57 | A17 L50 L51 L57 | L33 L34 L56 L57 L79 L80 | L50 L55 L56 L57 | L3 L4 L54 L55 L89 L90 | A12 A17 L50 L51 | A12 A17 L51 L59 | L32 L33 L57 L59 L78 L79 | L54 L55 L56 L89 L90 | L54 L55 L56 L57 | A17 L58 L59 L77 L78 | A12 A17 L58 L59 | A12 A17 L50 L59 | L54 L55 L57 L59 | L54 L56 L57 L97 L98 | L4 L5 L6 L7 L8 L9 L10 L11 L54 L56 L90 L91 L92 L93 L94 L95 L96 L97 | A12 A17 L51 L58 | L31 L32 L58 L59 L77 L78 | A17 L55 L58 L59 | L54 L55 L58 L59 | L11 L12 L56 L57 L97 L98 | A17 L50 L51 L69 L70 | A12 A17 L50 L51 | L24 L25 L26 L27 L28 L29 L30 L31 L51 L58 L70 L71 L72 L73 L74 L75 L76 L77 | A12 A17 L58 L59 | L54 L55 L58 L67 L68 | L54 L58 L59 L60 L99 | L12 L13 L57 L59 L98 L99 | A12 A17 L50 L58 | L23 L24 L50 L51 L69 L70 | L22 L23 L50 L55 L68 L69 | L21 L22 L54 L55 L67 L68 | L13 L14 L58 L59 L60 L99 | L14 L15 L16 L17 L18 L19 L20 L21 L54 L58 L60 L61 L62 L63 L64 L65 L66 L67
fillet "Fillet1" radius 4 72 edges at (-33.9411, 433.3832, 33.9411) (-59.6985, 481.3832, 8.1838) (-33.9411, 529.3832, 33.9411) (-59.6985, 577.3832, 8.1838) (-8.1838, 481.3832, 59.6985) (-8.1838, 577.3832, 59.6985) (-33.9411, 529.3832, -33.9411) (-33.9411, 433.3832, -33.9411) (-8.1838, 481.3832, -59.6985) (-8.1838, 577.3832, -59.6985) (33.9411, 529.3832, 33.9411) (33.9411, 433.3832, 33.9411) (59.6985, 481.3832, 8.1838) (59.6985, 577.3832, 8.1838) (59.6985, 577.3832, -8.1838) (33.9411, 529.3832, -33.9411) (59.6985, 481.3832, -8.1838) (33.9411, 433.3832, -33.9411) (-59.6985, 481.3832, -8.1838) (-59.6985, 577.3832, -8.1838) (8.1838, 481.3832, 59.6985) (8.1838, 577.3832, 59.6985) (8.1838, 481.3832, -59.6985) (8.1838, 577.3832, -59.6985) (33.9411, 542.6168, 33.9411) (59.6985, 494.6168, 8.1838) (33.9411, 446.6168, 33.9411) (59.6985, 398.6168, 8.1838) (-33.9411, 446.6168, 33.9411) (-33.9411, 542.6168, 33.9411) (-59.6985, 494.6168, 8.1838) (-59.6985, 398.6168, 8.1838) (33.9411, 446.6168, -33.9411) (8.1838, 494.6168, -59.6985) (33.9411, 542.6168, -33.9411) (8.1838, 398.6168, -59.6985) (-59.6985, 398.6168, -8.1838) (8.1838, 494.6168, 59.6985) (8.1838, 398.6168, 59.6985) (30.3905, 536, -37.4918) (56.1478, 488, -11.7344) (37.4918, 536, 30.3905) (37.4918, 440, 30.3905) (30.3905, 440, -37.4918) (37.4918, 536, -30.3905) (37.4918, 440, -30.3905) (59.6985, 494.6168, -8.1838) (59.6985, 398.6168, -8.1838) (11.7344, 488, -56.1478) (-33.9411, 542.6168, -33.9411) (-8.1838, 494.6168, -59.6985) (-8.1838, 398.6168, -59.6985) (-33.9411, 446.6168, -33.9411) (-59.6985, 494.6168, -8.1838) (-30.3905, 440, -37.4918) (-30.3905, 536, -37.4918) (-37.4918, 536, -30.3905) (-37.4918, 440, -30.3905) (-11.7344, 488, -56.1478) (-56.1478, 488, -11.7344) (-30.3905, 536, 37.4918) (-30.3905, 440, 37.4918) (-56.1478, 488, 11.7344) (-37.4918, 536, 30.3905) (-37.4918, 440, 30.3905) (-11.7344, 488, 56.1478) (-8.1838, 494.6168, 59.6985) (-8.1838, 398.6168, 59.6985) (30.3905, 536, 37.4918) (56.1478, 488, 11.7344) (30.3905, 440, 37.4918) (11.7344, 488, 56.1478)
fillet "Fillet2" radius 8 8 edges at (20.7107, 587, 50) (50, 587, 20.7107) (50, 587, -20.7107) (20.7107, 587, -50) (-20.7107, 587, -50) (-50, 587, -20.7107) (-50, 587, 20.7107) (-20.7107, 587, 50)
equation "d331 = ( 90 / 2 ) * 1 mm"
equation "d339 = 0.25 in + 0.3 mm"
equation "d340 = 4 mm + 0.3 mm"
equation "d539 = ( 48 / 2 ) * 1 mm"
equation "d540 = ( 36 / 2 ) * 1 mm"
